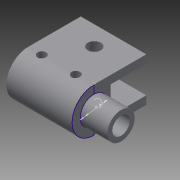
# Autodesk Inventor part: support_clip_base
Saved by Autodesk Inventor 2015 (Build 190159000, 159)
## iProperties
Created: 2017-10-02
Part Number: support_clip_base
Material: Generic
Document SubType Name: Modeling
Designer: Anshul
Density: 1 g/cm^3
Appearance: Default
Author: Anshul
Autodesk Inventor part; units mm, degrees
ref_plane "YZ Plane" through (0, 0, 0) normal (1, 0, 0) x (0, 1, 0)
ref_plane "XZ Plane" through (0, 0, 0) normal (0, 1, 0) x (-1, 0, 0)
ref_plane "XY Plane" through (0, 0, 0) normal (0, 0, 1) x (1, 0, 0)
sketch "Sketch1" plane through (0, 0, 0) normal (0, 1, 0) x (-1, 0, 0)
  line L0 (0, 0) -> (0, -280)
  line L1 (0, -280) -> (17, -280)
  line L2 (17, -280) -> (17, 0)
  line L3 (17, 0) -> (0, 0)
  line L4 (0, 0) -> (-10, 0)
  line L5 (-10, 0) -> (-10, -40)
  line L6 (-10, -40) -> (0, -40)
  line L7 (0, 0) -> (0, -125)
  line L8 (0, 0) -> (-70, 0)
  line L9 (0, -125) -> (0, -145)
  line L10 (0, -145) -> (0, -165)
  line L11 (-70, 0) -> (-70, -3.2)
  line L12 (-64.5656, 0) -> (-76.5656, 0)
  line L13 (-64.5656, 0) -> (-52.5656, 0)
  line L14 (-64.5656, -19.2569) -> (-76.5656, -19.2569)
  line L15 (-76.5656, -19.2569) -> (-76.5656, 0)
  line L16 (-64.5656, -19.2569) -> (-52.5656, -19.2569)
  line L17 (-52.5656, -19.2569) -> (-52.5656, 0)
  line L18 (-70, -3.2) -> (-76.5656, -3.2)
  line L19 (-70, -3.2) -> (-52.5656, -3.2)
  line L20 (-52.5656, -3.2) -> (-52.5656, -6.2)
  line L21 (-52.5656, -6.2) -> (-76.5656, -6.2)
  circle A0 centre (-64.5656, -12.2) radius 2.4
  line L22 (-64.5656, -12.2) -> (-64.5656, 0)
  line L23 (-64.5656, 0) -> (-71.5656, 0)
  line L24 (-64.5656, 0) -> (-57.5656, 0)
  circle A1 centre (-57.5656, 0) radius 1.55
  circle A2 centre (-70, 0) radius 1.55
  dimension "d0" = 280
  dimension "d1" = 17
  dimension "d2" = 280
  dimension "d3" = 10
  dimension "d4" = 40
  dimension "d5" = 125
  dimension "d6" = 70
  dimension "d7" = 20
  dimension "d8" = 20
  dimension "d11" = 3.2
  dimension "d12" = 12
  dimension "d16" = 3
  dimension "d18" = 4.8
  dimension "d28" = 7
  dimension "d29" = 7
  dimension "d30" = 3.1
  dimension "d31" = 3.1
  constraints: 50 end point, 16 point on line, 8 perpendicular, 3 centre point, 3 coincident, 3 vertical
  measures "d0" distance of L0.start L0.end
  measures "d1" distance of L0.end L1.end
  measures "d2" distance of L1.end L2.end
  measures "d3" distance of L0.start L4.end
  measures "d4" distance of L4.end L5.end
  measures "d5" distance of L0.start L7.end
  measures "d6" distance of L0.start L8.end
  measures "d7" distance of L7.end L9.end
  measures "d8" distance of L9.end L10.end
  measures "d11" distance of L11.start L11.end
  measures "d12" distance of L12.start L12.end
  measures "d16" distance of L19.end L20.end
  measures "d18" diameter of A0
  measures "d28" distance of L12.start L23.end
  measures "d29" distance of L12.start L24.end
  measures "d30" diameter of A1
  measures "d31" diameter of A2
extrude "Extrusion1" add sketch "Sketch1" along normal mid plane 16 contours L17 L19 L22 L8 A1 | A1 L8 | L17 L21 L22 L19 | L17 L16 L14 L15 L21 | L22 L21 L15 L18 L19 | L19 L11 A2 L8 L22 | L18 L15 L12 A2 L11 | A2 L11 L8 | A2 L12 L11 picked at (-58.5839, -0.1236)
extrude "Extrusion2" cut sketch "Sketch1" along normal mid plane 10 contours L17 L16 L14 L15 L21
sketch "Sketch2" plane through (76.5656, -8, 0) normal (1, 0, 0) x (0, 0, -1)
  arc A0 (0, 16) -> (0, 0) centre (0, 8) ccw
  arc A1 (0, 11.2) -> (0, 4.8) centre (0, 8) ccw
  line L0 (0, 16) -> (0, 0)
  line L1 (0, 0) -> (0, 16) projected
  circle A2 centre (0, 8) radius 3.2
  circle A3 centre (0, 8) radius 5
  dimension "d23" = 6.4
  dimension "d34" = 10
  constraints: 4 coincident, 4 point on circle, 3 centre point, 2 end point, 2 point on line, 1 collinear, 1 vertical alignment, 2 other
  measures "d23" diameter of A1
  measures "d34" diameter of A3
extrude "Extrusion3" add sketch "Sketch2" against normal blind 24 contours L0 A3 A0 | L0 A1 A3
extrude "Extrusion4" cut sketch "Sketch2" against normal blind 24 contours A2 L0
extrude "Extrusion5" cut sketch "Sketch1" along normal mid plane 20 contours A1 L8 | L8 A1 | A2 L11 L8 | L8 L12 A2 | A2 L12 L11
extrude "Extrusion6" add sketch "Sketch2" along normal blind 10 contours A3 L0 A2 | L0 A1 A3
body "Solid1"
